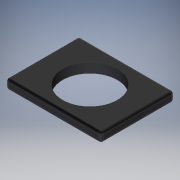
# Autodesk Inventor part: SyringeAttachment
Saved by Autodesk Inventor 2018 (Build 220112000, 112)
## iProperties
Created: 2018-01-14
Part Number: SyringeAttachment
Material: Generic
Document SubType Name: Modeling
Designer: reide
Density: 1 g/cm^3
Appearance: Default
Author: reide
Autodesk Inventor part; units mm, degrees
ref_plane "YZ Plane" through (0, 0, 0) normal (1, 0, 0) x (0, 1, 0)
ref_plane "XZ Plane" through (0, 0, 0) normal (0, 1, 0) x (-1, 0, 0)
ref_plane "XY Plane" through (0, 0, 0) normal (0, 0, 1) x (1, 0, 0)
sketch "Sketch1" plane through (0, 0, 0) normal (0, 0, 1) x (1, 0, 0)
  line L0 (-9.75, -4.725) -> (-9.75, 4.725) projected
  line L1 (9.75, 4.725) -> (9.75, -4.725) projected
  circle A0 centre (0, 0) radius 5.6
  line L2 (0, 0) -> (0, 7.5)
  line L3 (0, 0) -> (0, -7.5)
  line L4 (-9.75, 7.5) -> (9.75, 7.5)
  line L5 (9.75, 7.5) -> (9.75, -7.5)
  line L6 (9.75, -7.5) -> (-9.75, -7.5)
  line L7 (-9.75, -7.5) -> (-9.75, 7.5)
  point P0 (0, 0)
  dimension "d0" = 11.2
  dimension "d5" = 7.5
  dimension "d6" = 7.5
  constraints: 12 end point, 2 parallel, 2 vertical, 1 centre point, 1 coincident, 1 horizontal, 1 perpendicular
  measures "d0" diameter of A0
  measures "d5" distance of L2.start L2.end
  measures "d6" distance of L2.start L3.end
extrude "Extrusion1" add sketch "Sketch1" along normal blind 2 contours L0 L7 L4 L2 A0 L3 L6 | L3 A0 L2 L4 L5 L1 L6
fillet "Fillet1" radius 0.5 4 edges at (9.75, 7.5, 1) (-9.75, 7.5, 1) (-9.75, -7.5, 1) (9.75, -7.5, 1)
fillet "Fillet2" radius 0.5 16 edges at (-9.6036, 7.3536, 2) (-9.75, 0, 2) (-9.6036, -7.3536, 2) (0, -7.5, 2) (9.6036, -7.3536, 2) (9.75, 0, 2) (9.6036, 7.3536, 2) (0, 7.5, 2) (9.6036, 7.3536, 0) (9.75, 0, 0) (9.6036, -7.3536, 0) (0, -7.5, 0) (-9.6036, -7.3536, 0) (-9.75, 0, 0) (-9.6036, 7.3536, 0) (0, 7.5, 0)
body "Solid1"
